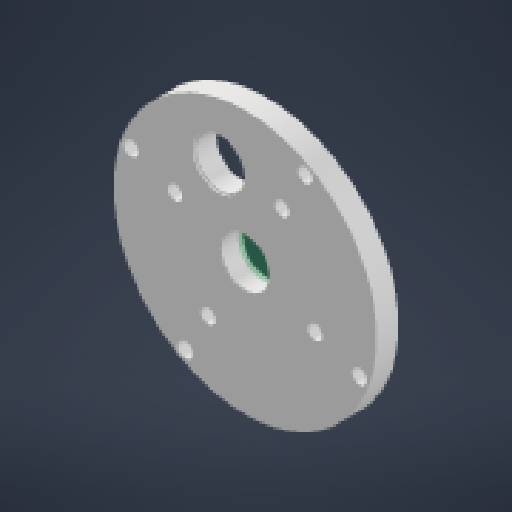
# Autodesk Inventor part: Inner_Pod_Holder
Saved by Autodesk Inventor 2024.2 (Build 282272000, 272)
## iProperties
Created: 2024-03-29
Part Number: Inner_Pod_Holder
Material: Generic
Document SubType Name: Modeling
Designer: warm
Density: 1 g/cm^3
Appearance: Default
Author: warm
Autodesk Inventor part; units mm, degrees
ref_plane "YZ Plane" through (0, 0, 0) normal (1, 0, 0) x (0, 1, 0)
ref_plane "XZ Plane" through (0, 0, 0) normal (0, 1, 0) x (-1, 0, 0)
ref_plane "XY Plane" through (0, 0, 0) normal (0, 0, 1) x (1, 0, 0)
ref_plane "Work Plane1" through (-28.6125, -68.0536, -6.35) normal (0, 0, -1) x (0, 1, 0)
sketch "Sketch1" plane through (0, 0, 0) normal (0, 0, 1) x (1, 0, 0)
  circle A0 centre (39.4411, 0) radius 38.42
  circle A1 centre (28.7179, -18.967) radius 2.975 construction
  circle A2 centre (18.97, 7.4611) radius 2.975 construction
  circle A3 centre (59.9122, -7.4611) radius 2.975 construction
  circle A4 centre (50.1643, 18.967) radius 2.875 construction
  circle A5 centre (39.4411, 0) radius 7
  circle A6 centre (31.7519, 21.0389) radius 7
  circle A7 centre (59.9122, -7.4611) radius 2.15
  circle A8 centre (50.1643, 18.967) radius 2.15
  circle A9 centre (18.97, 7.4611) radius 2.15
  circle A10 centre (28.7179, -18.967) radius 2.15
  point P0 (0, 0)
extrude "Extrusion1" add sketch "Sketch1" against normal up to surface (6.35 mm away)
ref_plane "Work Plane2" through (39.4411, 0, -4.95) normal (0, 0, -1) x (-0.4775827, -0.8785868, 0)
sketch "Sketch3" plane through (39.4411, 0, 0) normal (0, 0, 1) x (1, 0, 0)
  circle A0 centre (0, 0) radius 7.5 projected
  circle A1 centre (-7.6892, 21.0389) radius 7 construction
  circle A2 centre (-7.6892, 21.0389) radius 7.5
  point P0 (-39.4411, 0)
  dimension "d10" = 15
  constraints: 1 centre point, 1 coincident
  measures "d10" diameter of A2
extrude "Extrusion3" cut sketch "Sketch3" against normal blind 0.5 contours A2
sketch "Sketch5" plane through (39.4411, 0, 0) normal (0, 0, 1) x (1, 0, 0)
  circle A0 centre (0, 0) radius 7.3 construction
  circle A1 centre (0, 0) radius 7.5
  point P0 (-39.4411, 0)
  dimension "d11" = 15
  constraints: 1 centre point, 1 coincident
  measures "d11" diameter of A1
extrude "Extrusion4" cut sketch "Sketch5" against normal blind 0.05
sketch "Sketch6" plane through (39.4411, 0, 0) normal (0, 0, 1) x (1, 0, 0)
  circle A0 centre (20.4711, -7.4611) radius 2.975 construction
  circle A1 centre (10.7232, 18.967) radius 2.975 construction
  circle A2 centre (-20.4711, 7.4611) radius 2.975 construction
  circle A3 centre (-10.7232, -18.967) radius 2.975 construction
  line L0 (20.4711, -7.4611) -> (-20.4711, 7.4611) construction
  line L1 (-10.7232, -18.967) -> (10.7232, 18.967) construction
  circle A4 centre (17.4307, 30.8313) radius 2.15
  circle A5 centre (-17.4307, -30.8313) radius 2.15
  line L2 (17.4307, 30.8313) -> (-17.4307, -30.8313) construction
  circle A6 centre (0, 0) radius 38.42 construction
  circle A7 centre (33.2762, -12.1282) radius 2.15
  circle A8 centre (-33.2762, 12.1282) radius 2.15
  line L3 (33.2762, -12.1282) -> (-33.2762, 12.1282) construction
  point P0 (-39.4411, 0)
  dimension "d16" = 4.3
  dimension "d17" = 4.3
  dimension "d18" = 35.4175
  dimension "d19" = 35.4175
  dimension "d20" = 0
  dimension "d21" = 4.3
  dimension "d22" = 4.3
  dimension "d23" = 0
  dimension "d24" = 35.4175
  dimension "d25" = 35.4175
  dimension "d26" = 0
  constraints: 8 end point, 4 centre point
  measures "d16" diameter of A4
  measures "d17" diameter of A5
  measures "d18" distance of A6.centre L2.start
  measures "d19" distance of L2.end A6.centre
  measures "d20" distance between parallel lines of L1 L2
  measures "d21" diameter of A7
  measures "d22" diameter of A8
  measures "d23" distance between parallel lines of L0 L3
  measures "d24" distance of A6.centre L3.start
  measures "d25" distance of A6.centre L3.end
  measures "d26" distance from line of L0 L3.start
extrude "Extrusion5" cut sketch "Sketch6" against normal up to surface (6.35 mm away)
sketch "Sketch7" plane through (39.4411, 0, 0) normal (0, 0, 1) x (1, 0, 0)
  circle A0 centre (5.337, 26.1691) radius 2.15 construction
  circle A1 centre (-20.7154, 15.9087) radius 2.15 construction
  circle A2 centre (5.337, 26.1691) radius 4
  circle A3 centre (-20.7154, 15.9087) radius 4
  point P0 (-39.4411, 0)
  dimension "d29" = 8
  dimension "d30" = 8
  constraints: 2 centre point, 2 coincident
  measures "d29" diameter of A2
  measures "d30" diameter of A3
extrude "Extrusion6" cut sketch "Sketch7" against normal blind 3.81
sketch "Sketch8" plane through (44.7781, 26.1691, -3.81) normal (0, 0, 1) x (1, 0, 0)
  circle A0 centre (0, 0) radius 4 construction
  circle A1 centre (-26.0523, -10.2604) radius 4 construction
  circle A2 centre (0, 0) radius 2.15
  circle A3 centre (-26.0523, -10.2604) radius 2.15
  point P0 (-44.7781, -26.1691)
  dimension "d33" = 4.3
  dimension "d34" = 4.3
  constraints: 2 centre point, 2 coincident
  measures "d33" diameter of A2
  measures "d34" diameter of A3
extrude "Extrusion7" cut sketch "Sketch8" against normal through all
equation "\"d19\" = d18"
equation "\"d24\" = d18"
equation "\"d25\" = d18"
body "Solid1"
